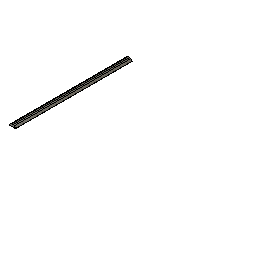
2020_Aluminum_Extrusion_Mounting_Spacer (Autodesk Fusion 360 design; units mm, degrees)
part number: 2026-08-29-22-42-17-088
Autodesk Fusion 360 part; units mm, degrees
sketch "Sketch1" plane through (0, -20, 0) normal (0, -1, 0) x (-1, 0, 0)
  line L0 (131.0061, 3.6) -> (128.8016, 3.6)
  arc A0 (126.6802, 4.4787) -> (128.8016, 3.6) centre (128.8016, 6.6) ccw
  line L1 (126.6802, 4.4787) -> (124.3794, 6.7796)
  arc A1 (124.9508, 8.0937) -> (124.3794, 6.7796) centre (124.9239, 7.3241) ccw
  line L2 (124.9508, 8.0937) -> (127.0686, 8.0198)
  arc A2 (127.0686, 8.0198) -> (127.3789, 8.3091) centre (127.0791, 8.3196) ccw
  line L3 (127.3789, 8.3091) -> (127.4033, 9.0087)
  arc A3 (127.4033, 9.0087) -> (126.6317, 9.8361) centre (126.6038, 9.0366) ccw
  line L4 (126.6317, 9.8361) -> (121.9736, 9.9988)
  arc A4 (121.9736, 9.9988) -> (119.905, 7.9302) centre (121.9038, 8) ccw
  line L5 (119.905, 7.9302) -> (120.0677, 3.2721)
  arc A5 (120.0677, 3.2721) -> (120.8951, 2.5005) centre (120.8672, 3.3) ccw
  line L6 (120.8951, 2.5005) -> (121.5947, 2.5249)
  arc A6 (121.5947, 2.5249) -> (121.884, 2.8352) centre (121.5842, 2.8247) ccw
  line L7 (121.884, 2.8352) -> (121.8101, 4.953)
  arc A7 (123.1243, 5.5244) -> (121.8101, 4.953) centre (122.5797, 4.9799) ccw
  line L8 (123.1243, 5.5244) -> (125.4251, 3.2236)
  arc A8 (126.3038, 1.1022) -> (125.4251, 3.2236) centre (123.3038, 1.1022) ccw
  line L9 (126.3038, 1.1022) -> (126.3038, -1.1022)
  arc A9 (125.4251, -3.2236) -> (126.3038, -1.1022) centre (123.3038, -1.1022) ccw
  line L10 (125.4251, -3.2236) -> (123.1243, -5.5244)
  arc A10 (121.8101, -4.953) -> (123.1243, -5.5244) centre (122.5797, -4.9799) ccw
  line L11 (121.8101, -4.953) -> (121.884, -2.8352)
  arc A11 (121.884, -2.8352) -> (121.5947, -2.5249) centre (121.5842, -2.8247) ccw
  line L12 (121.5947, -2.5249) -> (120.8951, -2.5005)
  arc A12 (120.8951, -2.5005) -> (120.0677, -3.2721) centre (120.8672, -3.3) ccw
  line L13 (120.0677, -3.2721) -> (119.905, -7.9302)
  arc A13 (119.905, -7.9302) -> (121.9736, -9.9988) centre (121.9038, -8) ccw
  line L14 (121.9736, -9.9988) -> (126.6317, -9.8361)
  arc A14 (126.6317, -9.8361) -> (127.4033, -9.0087) centre (126.6038, -9.0366) ccw
  line L15 (127.4033, -9.0087) -> (127.3789, -8.3091)
  arc A15 (127.3789, -8.3091) -> (127.0686, -8.0198) centre (127.0791, -8.3196) ccw
  line L16 (127.0686, -8.0198) -> (124.9508, -8.0937)
  arc A16 (124.3794, -6.7796) -> (124.9508, -8.0937) centre (124.9239, -7.3241) ccw
  line L17 (124.3794, -6.7796) -> (126.6802, -4.4787)
  arc A17 (128.8016, -3.6) -> (126.6802, -4.4787) centre (128.8016, -6.6) ccw
  line L18 (128.8016, -3.6) -> (131.0061, -3.6)
  arc A18 (133.1274, -4.4787) -> (131.0061, -3.6) centre (131.0061, -6.6) ccw
  line L19 (133.1274, -4.4787) -> (135.4283, -6.7796)
  arc A19 (134.8568, -8.0937) -> (135.4283, -6.7796) centre (134.8837, -7.3241) ccw
  line L20 (134.8568, -8.0937) -> (132.739, -8.0198)
  arc A20 (132.739, -8.0198) -> (132.4287, -8.3091) centre (132.7285, -8.3196) ccw
  line L21 (132.4287, -8.3091) -> (132.4043, -9.0087)
  arc A21 (132.4043, -9.0087) -> (133.1759, -9.8361) centre (133.2038, -9.0366) ccw
  line L22 (133.1759, -9.8361) -> (137.834, -9.9988)
  arc A22 (137.834, -9.9988) -> (139.9026, -7.9302) centre (137.9038, -8) ccw
  line L23 (139.9026, -7.9302) -> (139.7399, -3.2721)
  arc A23 (139.7399, -3.2721) -> (138.9125, -2.5005) centre (138.9404, -3.3) ccw
  line L24 (138.9125, -2.5005) -> (138.2129, -2.5249)
  arc A24 (138.2129, -2.5249) -> (137.9236, -2.8352) centre (138.2234, -2.8247) ccw
  line L25 (137.9236, -2.8352) -> (137.9975, -4.953)
  arc A25 (136.6834, -5.5244) -> (137.9975, -4.953) centre (137.2279, -4.9799) ccw
  line L26 (136.6834, -5.5244) -> (134.3825, -3.2236)
  arc A26 (133.5038, -1.1022) -> (134.3825, -3.2236) centre (136.5038, -1.1022) ccw
  line L27 (133.5038, -1.1022) -> (133.5038, 1.1022)
  arc A27 (134.3825, 3.2236) -> (133.5038, 1.1022) centre (136.5038, 1.1022) ccw
  line L28 (134.3825, 3.2236) -> (136.6834, 5.5244)
  arc A28 (137.9975, 4.953) -> (136.6834, 5.5244) centre (137.2279, 4.9799) ccw
  line L29 (137.9975, 4.953) -> (137.9236, 2.8352)
  arc A29 (137.9236, 2.8352) -> (138.2129, 2.5249) centre (138.2234, 2.8247) ccw
  line L30 (138.2129, 2.5249) -> (138.9125, 2.5005)
  arc A30 (138.9125, 2.5005) -> (139.7399, 3.2721) centre (138.9404, 3.3) ccw
  line L31 (139.7399, 3.2721) -> (139.9026, 7.9302)
  arc A31 (139.9026, 7.9302) -> (137.834, 9.9988) centre (137.9038, 8) ccw
  line L32 (137.834, 9.9988) -> (133.1759, 9.8361)
  arc A32 (133.1759, 9.8361) -> (132.4043, 9.0087) centre (133.2038, 9.0366) ccw
  line L33 (132.4043, 9.0087) -> (132.4287, 8.3091)
  arc A33 (132.4287, 8.3091) -> (132.739, 8.0198) centre (132.7285, 8.3196) ccw
  line L34 (132.739, 8.0198) -> (134.8568, 8.0937)
  arc A34 (135.4283, 6.7796) -> (134.8568, 8.0937) centre (134.8837, 7.3241) ccw
  line L35 (135.4283, 6.7796) -> (133.1274, 4.4787)
  arc A35 (131.0061, 3.6) -> (133.1274, 4.4787) centre (131.0061, 6.6) ccw
  circle A36 centre (129.9038, 0) radius 2.15
  arc A37 (124.9333, 7.594) -> (124.7329, 7.1331) centre (124.9239, 7.3241) ccw
  line L36 (127.0338, 4.8322) -> (124.7329, 7.1331)
  arc A38 (127.0338, 4.8322) -> (128.8016, 4.1) centre (128.8016, 6.6) ccw
  line L37 (131.0061, 4.1) -> (128.8016, 4.1)
  arc A39 (131.0061, 4.1) -> (132.7738, 4.8322) centre (131.0061, 6.6) ccw
  line L38 (135.0747, 7.1331) -> (132.7738, 4.8322)
  arc A40 (135.0747, 7.1331) -> (134.8743, 7.594) centre (134.8837, 7.3241) ccw
  line L39 (132.7565, 7.5201) -> (134.8743, 7.594)
  arc A41 (131.929, 8.2917) -> (132.7565, 7.5201) centre (132.7285, 8.3196) ccw
  line L40 (131.9046, 8.9912) -> (131.929, 8.2917)
  arc A42 (133.1584, 10.3358) -> (131.9046, 8.9912) centre (133.2038, 9.0366) ccw
  line L41 (137.8166, 10.4985) -> (133.1584, 10.3358)
  arc A43 (140.4023, 7.9128) -> (137.8166, 10.4985) centre (137.9038, 8) ccw
  line L42 (140.2396, 3.2546) -> (140.4023, 7.9128)
  arc A44 (138.895, 2.0008) -> (140.2396, 3.2546) centre (138.9404, 3.3) ccw
  line L43 (138.1955, 2.0252) -> (138.895, 2.0008)
  arc A45 (137.4239, 2.8527) -> (138.1955, 2.0252) centre (138.2234, 2.8247) ccw
  line L44 (137.4978, 4.9705) -> (137.4239, 2.8527)
  arc A46 (137.4978, 4.9705) -> (137.0369, 5.1709) centre (137.2279, 4.9799) ccw
  line L45 (134.736, 2.87) -> (137.0369, 5.1709)
  arc A47 (134.736, 2.87) -> (134.0038, 1.1022) centre (136.5038, 1.1022) ccw
  line L46 (134.0038, -1.1022) -> (134.0038, 1.1022)
  arc A48 (134.0038, -1.1022) -> (134.736, -2.87) centre (136.5038, -1.1022) ccw
  line L47 (137.0369, -5.1709) -> (134.736, -2.87)
  arc A49 (137.0369, -5.1709) -> (137.4978, -4.9705) centre (137.2279, -4.9799) ccw
  line L48 (137.4239, -2.8527) -> (137.4978, -4.9705)
  arc A50 (138.1955, -2.0252) -> (137.4239, -2.8527) centre (138.2234, -2.8247) ccw
  line L49 (138.895, -2.0008) -> (138.1955, -2.0252)
  arc A51 (140.2396, -3.2546) -> (138.895, -2.0008) centre (138.9404, -3.3) ccw
  line L50 (140.4023, -7.9128) -> (140.2396, -3.2546)
  arc A52 (137.8166, -10.4985) -> (140.4023, -7.9128) centre (137.9038, -8) ccw
  line L51 (133.1584, -10.3358) -> (137.8166, -10.4985)
  arc A53 (131.9046, -8.9912) -> (133.1584, -10.3358) centre (133.2038, -9.0366) ccw
  line L52 (131.929, -8.2917) -> (131.9046, -8.9912)
  arc A54 (132.7565, -7.5201) -> (131.929, -8.2917) centre (132.7285, -8.3196) ccw
  line L53 (134.8743, -7.594) -> (132.7565, -7.5201)
  arc A55 (134.8743, -7.594) -> (135.0747, -7.1331) centre (134.8837, -7.3241) ccw
  line L54 (132.7738, -4.8322) -> (135.0747, -7.1331)
  arc A56 (132.7738, -4.8322) -> (131.0061, -4.1) centre (131.0061, -6.6) ccw
  line L55 (128.8016, -4.1) -> (131.0061, -4.1)
  arc A57 (128.8016, -4.1) -> (127.0338, -4.8322) centre (128.8016, -6.6) ccw
  line L56 (124.7329, -7.1331) -> (127.0338, -4.8322)
  arc A58 (124.7329, -7.1331) -> (124.9333, -7.594) centre (124.9239, -7.3241) ccw
  line L57 (127.0512, -7.5201) -> (124.9333, -7.594)
  arc A59 (127.8786, -8.2917) -> (127.0512, -7.5201) centre (127.0791, -8.3196) ccw
  line L58 (127.903, -8.9912) -> (127.8786, -8.2917)
  arc A60 (126.6492, -10.3358) -> (127.903, -8.9912) centre (126.6038, -9.0366) ccw
  line L59 (121.9911, -10.4985) -> (126.6492, -10.3358)
  arc A61 (119.4053, -7.9128) -> (121.9911, -10.4985) centre (121.9038, -8) ccw
  line L60 (119.568, -3.2546) -> (119.4053, -7.9128)
  arc A62 (120.9126, -2.0008) -> (119.568, -3.2546) centre (120.8672, -3.3) ccw
  line L61 (121.6121, -2.0252) -> (120.9126, -2.0008)
  arc A63 (122.3837, -2.8527) -> (121.6121, -2.0252) centre (121.5842, -2.8247) ccw
  line L62 (122.3098, -4.9705) -> (122.3837, -2.8527)
  arc A64 (122.3098, -4.9705) -> (122.7707, -5.1709) centre (122.5797, -4.9799) ccw
  line L63 (125.0716, -2.87) -> (122.7707, -5.1709)
  arc A65 (125.0716, -2.87) -> (125.8038, -1.1022) centre (123.3038, -1.1022) ccw
  line L64 (125.8038, 1.1022) -> (125.8038, -1.1022)
  arc A66 (125.8038, 1.1022) -> (125.0716, 2.87) centre (123.3038, 1.1022) ccw
  line L65 (122.7707, 5.1709) -> (125.0716, 2.87)
  arc A67 (122.7707, 5.1709) -> (122.3098, 4.9705) centre (122.5797, 4.9799) ccw
  line L66 (122.3837, 2.8527) -> (122.3098, 4.9705)
  arc A68 (121.6121, 2.0252) -> (122.3837, 2.8527) centre (121.5842, 2.8247) ccw
  line L67 (120.9126, 2.0008) -> (121.6121, 2.0252)
  arc A69 (119.568, 3.2546) -> (120.9126, 2.0008) centre (120.8672, 3.3) ccw
  line L68 (119.4053, 7.9128) -> (119.568, 3.2546)
  arc A70 (121.9911, 10.4985) -> (119.4053, 7.9128) centre (121.9038, 8) ccw
  line L69 (126.6492, 10.3358) -> (121.9911, 10.4985)
  arc A71 (127.903, 8.9912) -> (126.6492, 10.3358) centre (126.6038, 9.0366) ccw
  line L70 (127.8786, 8.2917) -> (127.903, 8.9912)
  arc A72 (127.0512, 7.5201) -> (127.8786, 8.2917) centre (127.0791, 8.3196) ccw
  line L71 (124.9333, 7.594) -> (127.0512, 7.5201)
  line L72 (124.9333, 7.594) -> (134.8743, 7.594)
  dimension "d216" = 0.5
extrude "Extrude1" add sketch "Sketch1" against normal blind 9.5 contours A37 L36 A38 L37 A39 L38 A40 L39 A41 A72 L71 L72
extrude "Extrude2" add 1 faces at (-129.5364, -10.5, -6.4293) along direction (0, 1, 0) blind 352
extrude "Extrude3" cut 1 faces at (-129.5364, 341.5, -6.4293) along direction (0, -1, 0) blind 180.75
